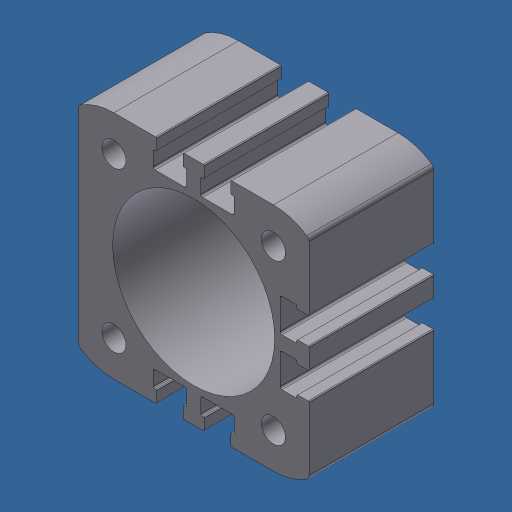
# Autodesk Inventor part: EXTRUSION,CYLINDER, ALUMINIUM, FESTO, 32MM
Saved by Autodesk Inventor 2024.3 (Build 283343000, 343)
## iProperties
Category: _
Manager: _
Control State: 0
Master: False
Checked Out: False
Part Number: EXTRUSION,CYLINDER, ALUMINIUM, FESTO, 32MM
Material: Aluminum, 6061-T6
Document SubType Name: Modeling
Created: 2019-07-31
Designer: -
Manufacturer: Standard
Standards Organization: Custom
Density: 2.71 g/cm^3
Mass: 71.3594 g
Surface Area: 129.472 cm^2
Volume: 26.3319 cm^3
Checked By: 00
Engr Approved By: _
User Status: Work In Process
Description: EXTRUSION, CYLINDER, ALUMINIUM, FESTO, 32MM
Mfg Approved By: -
Appearance: Aluminum (Flat)
Shininess: 64.0
Angle Display Precision: 2
Document Length Units: 11272
Document Angle Units: 11279
Document Time Units: 11290
Document Mass Units: 11286
Document Length Units Precision: 3
Document Angle Units Precision: 2
ILogicPurgeVersion: 2.2.20.20
Density: 0.0
Volumn: 0.0
Area: 0.0
PropertySet Name: Model Information
CN_MASS: 0.21
CN_SERVICEABLE: _
CL_runCount: 0
FIRST_DESCRIPTION: _
SECOND_DESCRIPTION: _
THIRD_DESCRIPTION: _
ModelCat: Uncategorized
Author: -
Subject: _
Revision Number: A
Keywords: -
Autodesk Inventor part; units mm, degrees
ref_plane "YZ Plane" through (0, 0, 0) normal (1, 0, 0) x (0, 1, 0)
ref_plane "XZ Plane" through (0, 0, 0) normal (0, 1, 0) x (-1, 0, 0)
ref_plane "XY Plane" through (0, 0, 0) normal (0, 0, 1) x (1, 0, 0)
sketch "Sketch1" plane through (0, 0, 0) normal (0, 0, 1) x (1, 0, 0)
  arc A0 (15.55, -15.95) -> (15.75, -15.75) centre (15.55, -15.75) ccw
  line L0 (15.75, -2.866) -> (15.75, -15.75)
  arc A1 (15.75, -2.866) -> (15.2982, -2.0297) centre (14.75, -2.866) ccw
  arc A2 (15.2982, -2.0297) -> (8.5, 0) centre (8.5, -12.4) ccw
  line L1 (0, 0) -> (8.5, 0)
  arc A3 (0, 0) -> (-0.2, -0.2) centre (0, -0.2) ccw
  line L2 (-0.2, -2.3) -> (-0.2, -0.2)
  arc A4 (-0.2, -2.3) -> (0, -2.5) centre (0, -2.3) ccw
  line L3 (0.3, -2.5) -> (0, -2.5)
  arc A5 (0.5, -2.7) -> (0.3, -2.5) centre (0.3, -2.7) ccw
  line L4 (0.5, -5.5) -> (0.5, -2.7)
  arc A6 (0.1, -5.9) -> (0.5, -5.5) centre (0.1, -5.5) ccw
  line L5 (-5.9, -5.9) -> (0.1, -5.9)
  arc A7 (-6.3, -5.5) -> (-5.9, -5.9) centre (-5.9, -5.5) ccw
  line L6 (-6.3, -2.7) -> (-6.3, -5.5)
  arc A8 (-6.1, -2.5) -> (-6.3, -2.7) centre (-6.1, -2.7) ccw
  line L7 (-5.8, -2.5) -> (-6.1, -2.5)
  arc A9 (-5.8, -2.5) -> (-5.6, -2.3) centre (-5.8, -2.3) ccw
  line L8 (-5.6, -0.2) -> (-5.6, -2.3)
  arc A10 (-5.6, -0.2) -> (-5.8, 0) centre (-5.8, -0.2) ccw
  line L9 (-9.7, 0) -> (-5.8, 0)
  arc A11 (-9.7, 0) -> (-9.9, -0.2) centre (-9.7, -0.2) ccw
  line L10 (-9.9, -2.3) -> (-9.9, -0.2)
  arc A12 (-9.9, -2.3) -> (-9.7, -2.5) centre (-9.7, -2.3) ccw
  line L11 (-9.4, -2.5) -> (-9.7, -2.5)
  arc A13 (-9.2, -2.7) -> (-9.4, -2.5) centre (-9.4, -2.7) ccw
  line L12 (-9.2, -5.5) -> (-9.2, -2.7)
  arc A14 (-9.6, -5.9) -> (-9.2, -5.5) centre (-9.6, -5.5) ccw
  line L13 (-15.6, -5.9) -> (-9.6, -5.9)
  arc A15 (-16, -5.5) -> (-15.6, -5.9) centre (-15.6, -5.5) ccw
  line L14 (-16, -2.7) -> (-16, -5.5)
  arc A16 (-15.8, -2.5) -> (-16, -2.7) centre (-15.8, -2.7) ccw
  line L15 (-15.5, -2.5) -> (-15.8, -2.5)
  arc A17 (-15.5, -2.5) -> (-15.3, -2.3) centre (-15.5, -2.3) ccw
  line L16 (-15.3, -0.2) -> (-15.3, -2.3)
  arc A18 (-15.3, -0.2) -> (-15.5, 0) centre (-15.5, -0.2) ccw
  line L17 (-24, 0) -> (-15.5, 0)
  arc A19 (-24, 0) -> (-30.7982, -2.0297) centre (-24, -12.4) ccw
  arc A20 (-30.7982, -2.0297) -> (-31.25, -2.866) centre (-30.25, -2.866) ccw
  line L18 (-31.25, -44.134) -> (-31.25, -2.866)
  arc A21 (-31.25, -44.134) -> (-30.7982, -44.9703) centre (-30.25, -44.134) ccw
  arc A22 (-30.7982, -44.9703) -> (-24, -47) centre (-24, -34.6) ccw
  line L19 (-15.5, -47) -> (-24, -47)
  arc A23 (-15.5, -47) -> (-15.3, -46.8) centre (-15.5, -46.8) ccw
  line L20 (-15.3, -44.7) -> (-15.3, -46.8)
  arc A24 (-15.3, -44.7) -> (-15.5, -44.5) centre (-15.5, -44.7) ccw
  line L21 (-15.8, -44.5) -> (-15.5, -44.5)
  arc A25 (-16, -44.3) -> (-15.8, -44.5) centre (-15.8, -44.3) ccw
  line L22 (-16, -41.5) -> (-16, -44.3)
  arc A26 (-15.6, -41.1) -> (-16, -41.5) centre (-15.6, -41.5) ccw
  line L23 (-9.6, -41.1) -> (-15.6, -41.1)
  arc A27 (-9.2, -41.5) -> (-9.6, -41.1) centre (-9.6, -41.5) ccw
  line L24 (-9.2, -44.3) -> (-9.2, -41.5)
  arc A28 (-9.4, -44.5) -> (-9.2, -44.3) centre (-9.4, -44.3) ccw
  line L25 (-9.7, -44.5) -> (-9.4, -44.5)
  arc A29 (-9.7, -44.5) -> (-9.9, -44.7) centre (-9.7, -44.7) ccw
  line L26 (-9.9, -46.8) -> (-9.9, -44.7)
  arc A30 (-9.9, -46.8) -> (-9.7, -47) centre (-9.7, -46.8) ccw
  line L27 (-5.8, -47) -> (-9.7, -47)
  arc A31 (-5.8, -47) -> (-5.6, -46.8) centre (-5.8, -46.8) ccw
  line L28 (-5.6, -44.7) -> (-5.6, -46.8)
  arc A32 (-5.6, -44.7) -> (-5.8, -44.5) centre (-5.8, -44.7) ccw
  line L29 (-6.1, -44.5) -> (-5.8, -44.5)
  arc A33 (-6.3, -44.3) -> (-6.1, -44.5) centre (-6.1, -44.3) ccw
  line L30 (-6.3, -41.5) -> (-6.3, -44.3)
  arc A34 (-5.9, -41.1) -> (-6.3, -41.5) centre (-5.9, -41.5) ccw
  line L31 (0.1, -41.1) -> (-5.9, -41.1)
  arc A35 (0.5, -41.5) -> (0.1, -41.1) centre (0.1, -41.5) ccw
  line L32 (0.5, -44.3) -> (0.5, -41.5)
  arc A36 (0.3, -44.5) -> (0.5, -44.3) centre (0.3, -44.3) ccw
  line L33 (0, -44.5) -> (0.3, -44.5)
  arc A37 (0, -44.5) -> (-0.2, -44.7) centre (0, -44.7) ccw
  line L34 (-0.2, -46.8) -> (-0.2, -44.7)
  arc A38 (-0.2, -46.8) -> (0, -47) centre (0, -46.8) ccw
  line L35 (8.5, -47) -> (0, -47)
  arc A39 (8.5, -47) -> (15.2982, -44.9703) centre (8.5, -34.6) ccw
  arc A40 (15.2982, -44.9703) -> (15.75, -44.134) centre (14.75, -44.134) ccw
  line L36 (15.75, -31.25) -> (15.75, -44.134)
  arc A41 (15.75, -31.25) -> (15.55, -31.05) centre (15.55, -31.25) ccw
  line L37 (13.45, -31.05) -> (15.55, -31.05)
  arc A42 (13.45, -31.05) -> (13.25, -31.25) centre (13.45, -31.25) ccw
  line L38 (13.25, -31.55) -> (13.25, -31.25)
  arc A43 (13.05, -31.75) -> (13.25, -31.55) centre (13.05, -31.55) ccw
  line L39 (10.25, -31.75) -> (13.05, -31.75)
  arc A44 (9.85, -31.35) -> (10.25, -31.75) centre (10.25, -31.35) ccw
  line L40 (9.85, -25.35) -> (9.85, -31.35)
  arc A45 (10.25, -24.95) -> (9.85, -25.35) centre (10.25, -25.35) ccw
  line L41 (13.05, -24.95) -> (10.25, -24.95)
  arc A46 (13.25, -25.15) -> (13.05, -24.95) centre (13.05, -25.15) ccw
  line L42 (13.25, -25.45) -> (13.25, -25.15)
  arc A47 (13.25, -25.45) -> (13.45, -25.65) centre (13.45, -25.45) ccw
  line L43 (15.55, -25.65) -> (13.45, -25.65)
  arc A48 (15.55, -25.65) -> (15.75, -25.45) centre (15.55, -25.45) ccw
  line L44 (15.75, -21.55) -> (15.75, -25.45)
  arc A49 (15.75, -21.55) -> (15.55, -21.35) centre (15.55, -21.55) ccw
  line L45 (13.45, -21.35) -> (15.55, -21.35)
  arc A50 (13.45, -21.35) -> (13.25, -21.55) centre (13.45, -21.55) ccw
  line L46 (13.25, -21.85) -> (13.25, -21.55)
  arc A51 (13.05, -22.05) -> (13.25, -21.85) centre (13.05, -21.85) ccw
  line L47 (10.25, -22.05) -> (13.05, -22.05)
  arc A52 (9.85, -21.65) -> (10.25, -22.05) centre (10.25, -21.65) ccw
  line L48 (9.85, -15.65) -> (9.85, -21.65)
  arc A53 (10.25, -15.25) -> (9.85, -15.65) centre (10.25, -15.65) ccw
  line L49 (13.05, -15.25) -> (10.25, -15.25)
  arc A54 (13.25, -15.45) -> (13.05, -15.25) centre (13.05, -15.45) ccw
  line L50 (13.25, -15.75) -> (13.25, -15.45)
  arc A55 (13.25, -15.75) -> (13.45, -15.95) centre (13.45, -15.75) ccw
  line L51 (15.55, -15.95) -> (13.45, -15.95)
  arc A56 (-7.75, -28) -> (-7.75, -19) centre (-7.75, -23.5) ccw
  arc A57 (-7.75, -19) -> (-7.75, -28) centre (-7.75, -23.5) ccw
  arc A58 (8.5, -11.75) -> (8.5, -2.75) centre (8.5, -7.25) ccw
  arc A59 (8.5, -2.75) -> (8.5, -11.75) centre (8.5, -7.25) ccw
  arc A60 (-24, -44.25) -> (-24, -35.25) centre (-24, -39.75) ccw
  arc A61 (-24, -35.25) -> (-24, -44.25) centre (-24, -39.75) ccw
  arc A62 (-28.4949, -7.0354) -> (-28.4949, -7.4646) centre (-24, -7.25) ccw
  line L52 (-28.4949, -7.0354) -> (-28, -6.1782)
  line L53 (-28, -6.1782) -> (-28, -5.1884)
  arc A63 (-27.7854, -4.8167) -> (-28, -5.1884) centre (-24, -7.25) ccw
  line L54 (-27.7854, -4.8167) -> (-26.9282, -4.3218)
  line L55 (-26.9282, -4.3218) -> (-26.4333, -3.4646)
  arc A64 (-26.0616, -3.25) -> (-26.4333, -3.4646) centre (-24, -7.25) ccw
  line L56 (-26.0616, -3.25) -> (-25.0718, -3.25)
  line L57 (-25.0718, -3.25) -> (-24.2146, -2.7551)
  arc A65 (-24, -2.75) -> (-24.2146, -2.7551) centre (-24, -7.25) ccw
  arc A66 (-23.7854, -2.7551) -> (-24, -2.75) centre (-24, -7.25) ccw
  line L58 (-23.7854, -2.7551) -> (-22.9282, -3.25)
  line L59 (-22.9282, -3.25) -> (-21.9384, -3.25)
  arc A67 (-21.5667, -3.4646) -> (-21.9384, -3.25) centre (-24, -7.25) ccw
  line L60 (-21.5667, -3.4646) -> (-21.0718, -4.3218)
  line L61 (-21.0718, -4.3218) -> (-20.2146, -4.8167)
  arc A68 (-20, -5.1884) -> (-20.2146, -4.8167) centre (-24, -7.25) ccw
  line L62 (-20, -5.1884) -> (-20, -6.1782)
  line L63 (-20, -6.1782) -> (-19.5051, -7.0354)
  arc A69 (-19.5051, -7.4646) -> (-19.5051, -7.0354) centre (-24, -7.25) ccw
  line L64 (-19.5051, -7.4646) -> (-20, -8.3218)
  line L65 (-20, -8.3218) -> (-20, -9.3116)
  arc A70 (-20.2146, -9.6833) -> (-20, -9.3116) centre (-24, -7.25) ccw
  line L66 (-20.2146, -9.6833) -> (-21.0718, -10.1782)
  line L67 (-21.0718, -10.1782) -> (-21.5667, -11.0354)
  arc A71 (-21.9384, -11.25) -> (-21.5667, -11.0354) centre (-24, -7.25) ccw
  line L68 (-21.9384, -11.25) -> (-22.9282, -11.25)
  line L69 (-22.9282, -11.25) -> (-23.7854, -11.7449)
  arc A72 (-24, -11.75) -> (-23.7854, -11.7449) centre (-24, -7.25) ccw
  arc A73 (-24.2146, -11.7449) -> (-24, -11.75) centre (-24, -7.25) ccw
  line L70 (-24.2146, -11.7449) -> (-25.0718, -11.25)
  line L71 (-25.0718, -11.25) -> (-26.0616, -11.25)
  arc A74 (-26.4333, -11.0354) -> (-26.0616, -11.25) centre (-24, -7.25) ccw
  line L72 (-26.4333, -11.0354) -> (-26.9282, -10.1782)
  line L73 (-26.9282, -10.1782) -> (-27.7854, -9.6833)
  arc A75 (-28, -9.3116) -> (-27.7854, -9.6833) centre (-24, -7.25) ccw
  line L74 (-28, -9.3116) -> (-28, -8.3218)
  line L75 (-28, -8.3218) -> (-28.4949, -7.4646)
  arc A76 (4.0051, -39.5354) -> (4.0051, -39.9646) centre (8.5, -39.75) ccw
  line L76 (4.0051, -39.5354) -> (4.5, -38.6782)
  line L77 (4.5, -38.6782) -> (4.5, -37.6884)
  arc A77 (4.7146, -37.3167) -> (4.5, -37.6884) centre (8.5, -39.75) ccw
  line L78 (4.7146, -37.3167) -> (5.5718, -36.8218)
  line L79 (5.5718, -36.8218) -> (6.0667, -35.9646)
  arc A78 (6.4384, -35.75) -> (6.0667, -35.9646) centre (8.5, -39.75) ccw
  line L80 (6.4384, -35.75) -> (7.4282, -35.75)
  line L81 (7.4282, -35.75) -> (8.2854, -35.2551)
  arc A79 (8.5, -35.25) -> (8.2854, -35.2551) centre (8.5, -39.75) ccw
  arc A80 (8.7146, -35.2551) -> (8.5, -35.25) centre (8.5, -39.75) ccw
  line L82 (8.7146, -35.2551) -> (9.5718, -35.75)
  line L83 (9.5718, -35.75) -> (10.5616, -35.75)
  arc A81 (10.9333, -35.9646) -> (10.5616, -35.75) centre (8.5, -39.75) ccw
  line L84 (10.9333, -35.9646) -> (11.4282, -36.8218)
  line L85 (11.4282, -36.8218) -> (12.2854, -37.3167)
  arc A82 (12.5, -37.6884) -> (12.2854, -37.3167) centre (8.5, -39.75) ccw
  line L86 (12.5, -37.6884) -> (12.5, -38.6782)
  line L87 (12.5, -38.6782) -> (12.9949, -39.5354)
  arc A83 (12.9949, -39.9646) -> (12.9949, -39.5354) centre (8.5, -39.75) ccw
  line L88 (12.9949, -39.9646) -> (12.5, -40.8218)
  line L89 (12.5, -40.8218) -> (12.5, -41.8116)
  arc A84 (12.2854, -42.1833) -> (12.5, -41.8116) centre (8.5, -39.75) ccw
  line L90 (12.2854, -42.1833) -> (11.4282, -42.6782)
  line L91 (11.4282, -42.6782) -> (10.9333, -43.5354)
  arc A85 (10.5616, -43.75) -> (10.9333, -43.5354) centre (8.5, -39.75) ccw
  line L92 (10.5616, -43.75) -> (9.5718, -43.75)
  line L93 (9.5718, -43.75) -> (8.7146, -44.2449)
  arc A86 (8.5, -44.25) -> (8.7146, -44.2449) centre (8.5, -39.75) ccw
  arc A87 (8.2854, -44.2449) -> (8.5, -44.25) centre (8.5, -39.75) ccw
  line L94 (8.2854, -44.2449) -> (7.4282, -43.75)
  line L95 (7.4282, -43.75) -> (6.4384, -43.75)
  arc A88 (6.0667, -43.5354) -> (6.4384, -43.75) centre (8.5, -39.75) ccw
  line L96 (6.0667, -43.5354) -> (5.5718, -42.6782)
  line L97 (5.5718, -42.6782) -> (4.7146, -42.1833)
  arc A89 (4.5, -41.8116) -> (4.7146, -42.1833) centre (8.5, -39.75) ccw
  line L98 (4.5, -41.8116) -> (4.5, -40.8218)
  line L99 (4.5, -40.8218) -> (4.0051, -39.9646)
  circle A90 centre (-7.75, -23.5) radius 16.5
  dimension "d2" = 33
  constraints: 200 end point, 180 point on circle, 91 centre point, 5 coincident
  measures "d2" diameter of A90
extrude "FESTO, 32MM" add sketch "Sketch1" along normal blind 25.4 contours L51 A55 L50 A54 L49 A53 L48 A52 L47 A51 L46 A50 L45 A49 L44 A48 L43 A47 L42 A46 L41 A45 L40 A44 L39 A43 L38 A42 L37 A41 L36 A40 A39 L35 A38 L34 A37 L33 A36 L32 A35 L31 A34 L30 A33 L29 A32 L28 A31 L27 A30 L26 A29 L25 A28 L24 A27 L23 A26 L22 A25 L21 A24 L20 A23 L19 A22 A21 L18 A20 A19 L17 A18 L16 A17 L15 A16 L14 A15 L13 A14 L12 A13 L11 A12 L10 A11 L9 A10 L8 A9 L7 A8 L6 A7 L5 A6 L4 A5 L3 A4 L2 A3 L1 A2 A1 L0 A0 | A59 A58 | A61 A60 | L52 L53 A63 L54 L55 A64 L56 L57 A65 A66 L58 L59 A67 L60 L61 A68 L62 L63 A69 L64 L65 A70 L66 L67 A71 L68 L69 A72 A73 L70 L71 A74 L72 L73 A75 L74 L75 A62 | L76 L77 A77 L78 L79 A78 L80 L81 A79 A80 L82 L83 A81 L84 L85 A82 L86 L87 A83 L88 L89 A84 L90 L91 A85 L92 L93 A86 A87 L94 L95 A88 L96 L97 A89 L98 L99 A76
hole "Hole1" at (8.5, -7.25, 0) at (-24, -7.25, 0) at (-24, -39.75, 0) at (8.5, -39.75, 0) direction (0, 0, 1) diameter 4.91 end through all
